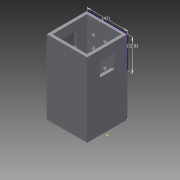
# Autodesk Inventor part: CraneArmBase
Saved by Autodesk Inventor 2015 (Build 190159000, 159)
## iProperties
Created: 2016-03-24
Part Number: CraneArmBase
Material: Generic
Document SubType Name: Modeling
Designer: Hatch
Density: 1 g/cm^3
Appearance: Default
Author: Hatch
Autodesk Inventor part; units mm, degrees
ref_plane "YZ Plane" through (0, 0, 0) normal (1, 0, 0) x (0, 1, 0)
ref_plane "XZ Plane" through (0, 0, 0) normal (0, 1, 0) x (-1, 0, 0)
ref_plane "XY Plane" through (0, 0, 0) normal (0, 0, 1) x (1, 0, 0)
sketch "Sketch1" plane through (0, 0, 0) normal (0, 1, 0) x (-1, 0, 0)
  line L0 (-21, 21) -> (21, 21)
  line L1 (21, 21) -> (21, -21)
  line L2 (21, -21) -> (-21, -21)
  line L3 (-21, -21) -> (-21, 21)
  line L4 (-21, 21) -> (21, -21) construction
  line L5 (21, 21) -> (-21, -21) construction
  point P0 (0, 0)
  dimension "d0" = 42
  dimension "d1" = 42
  constraints: 12 end point, 2 midpoint, 2 parallel, 1 horizontal, 1 perpendicular
  measures "d0" distance of L1.end L2.end
  measures "d1" distance of L0.end L1.end
extrude "Extrusion1" add sketch "Sketch1" along normal blind 101.6
sketch "Sketch2" plane through (0, 101.6, 0) normal (0, 1, 0) x (1, 0, 0)
  line L0 (21, 21) -> (-21, 21) projected
  line L1 (0, 21) -> (0, 18)
  line L2 (0, 18) -> (-18, 18)
  line L3 (-18, 18) -> (18, 18)
  line L4 (18, 18) -> (18, 14)
  line L5 (18, 14) -> (-18, 14)
  line L6 (-18, 14) -> (-18, 18)
  line L7 (21, -21) -> (21, 21) projected
  point P0 (0, 0)
  dimension "d4" = 3
  dimension "d5" = 18
  dimension "d6" = 36
  dimension "d7" = 4
  constraints: 12 end point, 2 parallel, 2 perpendicular, 1 horizontal, 1 midpoint, 1 vertical
  measures "d4" distance of L1.start L1.end
  measures "d5" distance of L1.end L2.end
  measures "d6" distance of L2.end L3.end
  measures "d7" distance of L3.end L4.end
extrude "Extrusion2" cut sketch "Sketch2" against normal through all
sketch "Sketch3" plane through (21, 0, -21) normal (0, 0, -1) x (-1, 0, 0)
  line L0 (0, 101.6) -> (42, 101.6) projected
  line L1 (21, 101.6) -> (21, 0)
  line L2 (21, 50.8) -> (39, 50.8)
  line L3 (39, 101.6) -> (39, 0) projected
  circle A0 centre (21, 50.8) radius 2.125
  dimension "d10" = 4.25
  constraints: 4 end point, 3 midpoint, 1 centre point, 1 coincident, 1 vertical
  measures "d10" diameter of A0
extrude "Extrusion3" cut sketch "Sketch3" against normal blind 3 contours A0 L2 L1 | L1 A0 | L2 A0 L1
pattern_linear "Rectangular Pattern1" count 2 spacing 12 along (-1, 0, 0) count 4 spacing 12 along (0, 1, 0) of "Extrusion3"
pattern_linear "Rectangular Pattern2" count 4 spacing 12 along (0, 1, 0) count 2 spacing 12 along (1, 0, 0) of "Extrusion3"
sketch "Sketch4" plane through (-21, 0, -21) normal (-1, 0, 0) x (0, 0, 1)
  line L0 (42, 0) -> (42, 101.6) projected
  line L1 (7, 101.6) -> (7, 0) projected
  line L2 (7, 72.8791) -> (9, 72.8791)
  line L3 (0, 101.6) -> (42, 101.6) projected
  line L4 (19.3629, 101.6) -> (19.3629, 91.6)
  line L5 (21, 91.6) -> (28.5, 91.6)
  line L6 (28.5, 91.6) -> (28.5, 76.6)
  line L7 (28.5, 76.6) -> (13.5, 76.6)
  line L8 (13.5, 76.6) -> (13.5, 91.6)
  line L9 (13.5, 91.6) -> (21, 91.6)
  point P0 (21, 0)
  dimension "d25" = 2
  dimension "d26" = 10
  dimension "d27" = 91.6
  dimension "d30" = 7.5
  dimension "d31" = 15
  dimension "d32" = 15
  dimension "d33" = 15
  constraints: 14 end point, 3 point on line, 2 perpendicular, 1 collinear, 1 horizontal, 1 vertical
  measures "d25" distance of L2.start L2.end
  measures "d26" distance of L4.start L4.end
  measures "d27" distance of point (21, 0) L5.start
  measures "d30" distance of L5.start L5.end
  measures "d31" distance of L5.end L6.end
  measures "d32" distance of L6.end L7.end
  measures "d33" distance of L7.end L8.end
extrude "Extrusion4" cut sketch "Sketch4" against normal through all
sketch "Sketch5" plane through (21, 0, -21) normal (0, 0, -1) x (-1, 0, 0)
  point P0 (21, 0)
sketch "Sketch6" plane through (0, 0, 0) normal (0, -1, 0) x (1, 0, 0)
  line L0 (-18, -14) -> (18, -14)
  line L1 (18, -14) -> (18, -18)
  line L2 (18, -18) -> (-18, -18)
  line L3 (-18, -18) -> (-18, -14)
  line L4 (-18, -14) -> (18, -18) construction
  line L5 (18, -14) -> (-18, -18) construction
  point P0 (0, 0)
  point P1 (0, -16)
  constraints: 12 end point, 2 midpoint, 2 parallel, 1 horizontal, 1 perpendicular
extrude "Extrusion5" add sketch "Sketch6" against normal blind 45
sketch "Sketch7" plane through (0, 101.6, 0) normal (0, 1, 0) x (1, 0, 0)
  line L0 (-18, 18) -> (-18, -18)
  line L1 (-21, -21) -> (21, -21) projected
  line L2 (-18, -18) -> (18, -18)
  line L3 (18, 18) -> (18, 14) projected
  line L4 (18, -18) -> (18, 18)
  line L5 (18, 18) -> (-18, 18)
  point P0 (0, 0)
  dimension "d38" = 36
  dimension "d39" = 36
  constraints: 8 end point, 1 horizontal, 1 perpendicular
  measures "d38" distance of L0.start L0.end
  measures "d39" distance of L0.end L2.end
extrude "Extrusion6" cut sketch "Sketch7" against normal through all
sketch "Sketch8" plane through (21, 0, -21) normal (0, 0, -1) x (-1, 0, 0)
  line L0 (-0.2731, 24.5) -> (42.2731, 24.5)
  line L1 (42.2731, 24.5) -> (42.2731, -24.5)
  line L2 (42.2731, -24.5) -> (-0.2731, -24.5)
  line L3 (-0.2731, -24.5) -> (-0.2731, 24.5)
  line L4 (-0.2731, 24.5) -> (42.2731, -24.5) construction
  line L5 (42.2731, 24.5) -> (-0.2731, -24.5) construction
  point P0 (21, 0)
  dimension "d42" = 49
  constraints: 12 end point, 2 midpoint, 2 parallel, 1 horizontal, 1 perpendicular
  measures "d42" distance of L0.end L1.end
extrude "Extrusion7" cut sketch "Sketch8" against normal through all
sketch "Sketch9" plane through (21, 101.6, -21) normal (0, 0, -1) x (-1, 0, 0)
  circle A0 centre (33, -26.8) radius 2.125 projected
  circle A1 centre (33, -38.8) radius 2.125 projected
  line L0 (33, -26.8) -> (33, -38.8)
  line L1 (33, -32.8) -> (42, -32.8)
  line L2 (42, -77.1) -> (42, 0) projected
  line L3 (42, -32.8) -> (0, -32.8)
  line L4 (0, -32.8) -> (0, 0)
  line L5 (0, 0) -> (42, 0)
  line L6 (42, 0) -> (42, -32.8)
  circle A2 centre (21, -26.8) radius 2.125 projected
  line L7 (21, -32.8) -> (21, -26.8)
  line L8 (42, -77.1) -> (39, -77.1)
  line L9 (0, -77.1) -> (42, -77.1) projected
  point P0 (21, -101.6)
  dimension "d45" = 42
  dimension "d46" = 32.8
  constraints: 16 end point, 2 horizontal, 2 midpoint, 2 parallel, 2 vertical, 1 collinear, 1 perpendicular, 1 point on line
  measures "d45" distance of L4.end L5.end
  measures "d46" distance of L3.end L4.end
body "Solid1"
